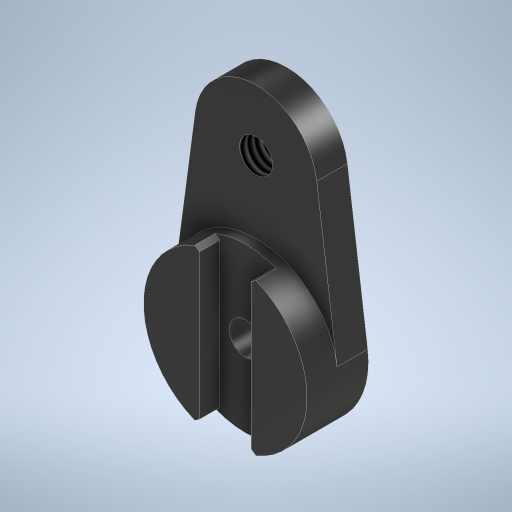
# Autodesk Inventor part: ICutShortCrankFrame
Saved by Autodesk Inventor 2024.2 (Build 282272000, 272)
## iProperties
Created: 2024-01-04
Part Number: ICutShortCrankFrame
Material: Aluminum 7075
Document SubType Name: Modeling
Designer: Masato Kubotera
Density: 2.81 g/cm^3
Appearance: Glossy - Black
Vendor: meviy
Mass: 3.8669 g
Surface Area: 11.8236 cm^2
Volume: 1.37612 cm^3
Author: Masato Kubotera
Autodesk Inventor part; units mm, degrees
ref_plane "YZ Plane" through (0, 0, 0) normal (1, 0, 0) x (0, 1, 0)
ref_plane "XZ Plane" through (0, 0, 0) normal (0, 1, 0) x (-1, 0, 0)
ref_plane "XY Plane" through (0, 0, 0) normal (0, 0, 1) x (1, 0, 0)
sketch "Sketch1" plane through (0, 0, 0) normal (1, 0, 0) x (0, 1, 0)
  circle A0 centre (0, 0) radius 8
  line L0 (0, 15) -> (0, 0) construction
  arc A1 (5.9464, 15.8) -> (-5.9464, 15.8) centre (0, 15) ccw
  line L1 (-7.9286, 1.0667) -> (-5.9464, 15.8)
  line L2 (7.9286, 1.0667) -> (5.9464, 15.8)
  line L3 (-2.5, 7.5993) -> (-2.5, -7.5993) construction
  line L4 (2.5, 7.5993) -> (2.5, -7.5993) construction
  line L5 (-2.525, 7.5911) -> (-2.525, -7.5911)
  line L6 (2.525, 7.5911) -> (2.525, -7.5911)
  line L7 (-7.5993, -2.5) -> (7.5993, -2.5) construction
  line L8 (-7.5911, -2.525) -> (7.5911, -2.525)
  line L9 (-7.5993, 2.5) -> (7.5993, 2.5) construction
  line L10 (-7.5911, 2.525) -> (7.5911, 2.525)
  point P0 (2.525, -7.5911)
  point P1 (2.525, 7.5911)
  point P2 (2.525, 2.525)
  point P3 (2.525, -2.525)
  point P4 (-2.525, 2.525)
  point P5 (-7.5911, 2.525)
  point P6 (-7.5911, -2.525)
  point P7 (-2.525, -2.525)
  dimension "d0" = 16
  dimension "d1" = 15
  dimension "d2" = 12
  dimension "d3" = 5
  dimension "d4" = 0.025
  dimension "d30" = 90
  constraints: 22 end point, 7 point on circle, 6 symmetric about line, 3 coincident, 2 centre point, 2 tangent, 2 vertical, 1 parallel, 13 other
  measures "d0" diameter of A0
  measures "d1" distance of L0.start L0.end
  measures "d2" diameter of A1
  measures "d3" distance between parallel lines of L4 L3
  measures "d4" distance between parallel lines of L4 L6
extrude "Extrusion1" add sketch "Sketch1" against normal blind 6
extrude "Extrusion2" cut sketch "Sketch1" against normal blind 3 contours A0 L1 A1 L2
extrude "Extrusion3" cut sketch "Sketch1" against normal blind 2 contours A0 L5 L8 L6 | L8 L5 L10 L6 | L6 L10 L5 A0
hole "M4" at (0, 0, 15) direction (-1, 0, 0) diameter 3.242 end through all thread size "M4x0.7" class "6H" standard "ANSI Metric M Profile"
hole "Phi3.2" at (0, 0, 0) direction (-1, 0, 0) diameter 3.2 end through all
chamfer "C0.5" distance 0.5 angle 45 4 edges at (-1, -2.525, -7.5911) (-1, 2.525, -7.5911) (-1, -2.525, 7.5911) (-1, 2.525, 7.5911)
body "Solid1"
